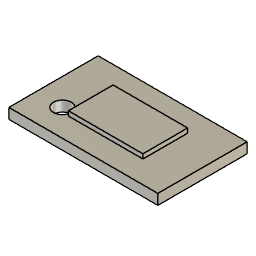
fixture-multi-tool (Autodesk Fusion 360 design; units mm, degrees)
part number: 2026-04-07-16-37-38-483
Autodesk Fusion 360 part; units mm, degrees
sketch "sketch_base_outline" plane through (0, 0, 0) normal (0, 0, 1) x (1, 0, 0)
  line L0 (0, 0) -> (100, 0)
  line L1 (100, 0) -> (100, 60)
  line L2 (100, 60) -> (0, 60)
  line L3 (0, 60) -> (0, 0)
extrude "Extrude1" add sketch "sketch_base_outline" along normal blind 10
sketch "sketch_center_pocket" plane through (0, 0, 10) normal (0, 0, 1) x (1, 0, 0)
  line L0 (0, 60) -> (0, 0)
  line L1 (0, 0) -> (100, 0)
  line L2 (100, 0) -> (100, 60)
  line L3 (100, 60) -> (0, 60)
  line L4 (25, 15) -> (75, 15)
  line L5 (75, 15) -> (75, 45)
  line L6 (75, 45) -> (25, 45)
  line L7 (25, 45) -> (25, 15)
extrude "center_pocket" cut sketch "sketch_center_pocket" against normal blind 3
sketch "sketch_bore_hole" plane through (0, 0, 10) normal (0, 0, 1) x (1, 0, 0)
  line L0 (75, 45) -> (25, 45)
  line L1 (25, 45) -> (25, 15)
  line L2 (25, 15) -> (75, 15)
  line L3 (75, 15) -> (75, 45)
  circle A0 centre (18, 18) radius 6
extrude "bore_hole" cut sketch "sketch_bore_hole" against normal blind 10 contours A0
equation "d3 = -( 3 mm )"
equation "d5 = -( 10 mm )"
named bodies: "fixture_plate"
